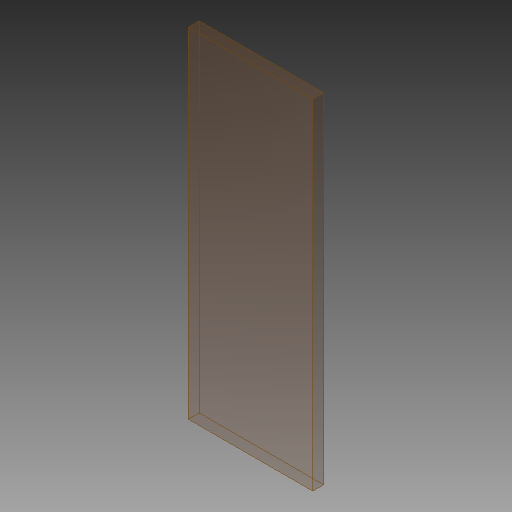
# Autodesk Inventor part: saw blade poly no hole mount
Saved by Autodesk Inventor 2019 (Build 230136000, 136)
## iProperties
Created: 2018-01-22
Part Number: saw blade poly no hole mount
Material: Polycarbonate, Smoke
Document SubType Name: Modeling
Designer: Administrator
Density: 1.2 g/cm^3
Appearance: Polycarbonate - Smoked
Author: Administrator
Autodesk Inventor part; units mm, degrees
ref_plane "YZ Plane" through (0, 0, 0) normal (1, 0, 0) x (0, 1, 0)
ref_plane "XZ Plane" through (0, 0, 0) normal (0, 1, 0) x (-1, 0, 0)
ref_plane "XY Plane" through (0, 0, 0) normal (0, 0, 1) x (1, 0, 0)
sketch "Sketch1" plane through (0, 0, 0) normal (0, 0, 1) x (1, 0, 0)
  line L0 (0, 0) -> (72.1614, 0)
  line L1 (72.1614, 0) -> (72.1614, 196.85)
  line L2 (72.1614, 196.85) -> (0, 196.85)
  line L3 (0, 196.85) -> (0, 0)
  dimension "d0" = 72.1614
  dimension "d1" = 196.85
  constraints: 8 end point, 2 parallel, 1 horizontal, 1 perpendicular
  measures "d0" distance of L0.start L0.end
  measures "d1" distance of L0.end L1.end
extrude "Extrusion1" add sketch "Sketch1" along normal blind 6.35
body "Solid1"
